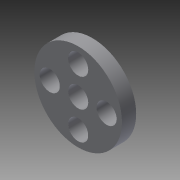
# Autodesk Inventor part: Picker
Saved by Autodesk Inventor 2015 (Build 190159000, 159)
## iProperties
Created: 2016-04-24
Part Number: Picker
Material: Generic
Document SubType Name: Modeling
Designer: Hatch
Density: 1 g/cm^3
Appearance: Default
Author: Hatch
Autodesk Inventor part; units mm, degrees
ref_plane "YZ Plane" through (0, 0, 0) normal (1, 0, 0) x (0, 1, 0)
ref_plane "XZ Plane" through (0, 0, 0) normal (0, 1, 0) x (-1, 0, 0)
ref_plane "XY Plane" through (0, 0, 0) normal (0, 0, 1) x (1, 0, 0)
sketch "Sketch1" plane through (0, 0, 0) normal (0, 1, 0) x (-1, 0, 0)
  line L0 (0, 0) -> (0, -19.05)
  circle A0 centre (0, -19.05) radius 4
  circle A1 centre (0, 0) radius 25
  dimension "d0" = 19.05
  dimension "d1" = 8
  dimension "d2" = 50
  constraints: 2 centre point, 2 coincident, 2 end point, 1 vertical
  measures "d0" distance of L0.start L0.end
  measures "d1" diameter of A0
  measures "d2" diameter of A1
extrude "Extrusion1" add sketch "Sketch1" along normal blind 5 contours A0 | A1
sketch "Sketch2" plane through (0, 5, 0) normal (0, 1, 0) x (1, 0, 0)
  line L0 (0, 0) -> (0, 19.05)
  circle A0 centre (0, 19.05) radius 3.9
  dimension "d5" = 19.05
  dimension "d6" = 7.8
  constraints: 2 end point, 1 centre point, 1 coincident, 1 vertical
  measures "d5" distance of L0.start L0.end
  measures "d6" diameter of A0
extrude "Extrusion2" add sketch "Sketch2" along normal blind 9
sketch "Sketch4" plane through (0, 5, 0) normal (0, 1, 0) x (1, 0, 0)
  circle A0 centre (0, 0) radius 9.25
  dimension "d9" = 18.5
  constraints: 1 centre point, 1 coincident
  measures "d9" diameter of A0
extrude "Extrusion3" cut sketch "Sketch4" against normal blind 2
sketch "Sketch5" plane through (0, 3, 0) normal (0, 1, 0) x (1, 0, 0)
  line L0 (0, 0) -> (0, -6)
  circle A0 centre (0, -6) radius 2.125
  dimension "d12" = 6
  dimension "d13" = 4.25
  constraints: 2 end point, 1 centre point, 1 coincident, 1 vertical
  measures "d12" distance of L0.start L0.end
  measures "d13" diameter of A0
extrude "Extrusion4" cut sketch "Sketch5" against normal through all
pattern_circular "Circular Pattern1" count 4 over 360 about axis through (0, 0, 0) along (0, 1, 0) of "Extrusion4"
sketch "Sketch6" plane through (0, 0, 0) normal (0, -1, 0) x (1, 0, 0)
  circle A0 centre (0, 0) radius 9
  circle A1 centre (0, 0) radius 2.125
  dimension "d19" = 18
  dimension "d20" = 4.25
  constraints: 2 centre point, 2 coincident
  measures "d19" diameter of A0
  measures "d20" diameter of A1
extrude "Extrusion5" cut sketch "Sketch6" against normal through all contours A1
sketch "Sketch7" plane through (0, 5, 0) normal (0, 1, 0) x (1, 0, 0)
  point P0 (0, 0)
sketch "Sketch8" plane through (0, 5, 0) normal (0, 1, 0) x (1, 0, 0)
  circle A0 centre (0, 0) radius 9.25
  circle A1 centre (0, 0) radius 25
  constraints: 2 centre point, 2 coincident
extrude "Extrusion6" cut sketch "Sketch8" along normal through all both and the other way through all
body "Solid1"
